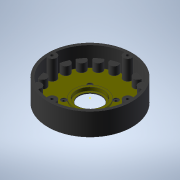
# Autodesk Inventor part: Część8
Saved by Autodesk Inventor 2021 (Build 250183000, 183)
## iProperties
Created: 2022-08-30
Part Number: Część8
Material: Ogólny
Document SubType Name: Modeling
Designer: MicnedSQ
Density: 1 g/cm^3
Appearance: Domyślna
Author: MicnedSQ
## iProperties of the stored document _Drukowanie 3D.ipt
Created: 2022-09-01
Part Number: _Drukowanie 3D
Material: Ogólny
Document SubType Name: Modeling
Designer: MicnedSQ
Density: 1 g/cm^3
Appearance: Domyślna
Author: MicnedSQ
Autodesk Inventor part; units mm, degrees
ref_plane "YZ Plane" through (0, 0, 0) normal (1, 0, 0) x (0, 1, 0)
ref_plane "XZ Plane" through (0, 0, 0) normal (0, 1, 0) x (-1, 0, 0)
ref_plane "XY Plane" through (0, 0, 0) normal (0, 0, 1) x (1, 0, 0)
sketch "Szkic1" plane through (0, 0, 0) normal (0, 1, 0) x (-1, 0, 0)
  circle A0 centre (0, 0) radius 50
  dimension "d1" = 100
  constraints: 1 centre point
  measures "d1" diameter of A0
extrude "Wyciągnięcie proste1" add sketch "Szkic1" along normal blind 5
sketch "Szkic2" plane through (0, 5, 0) normal (0, 1, 0) x (1, 0, 0)
  circle A0 centre (0, 0) radius 13.5
  dimension "d4" = 27
  constraints: 1 centre point, 1 coincident
  measures "d4" diameter of A0
extrude "Wyciągnięcie proste2" cut sketch "Szkic2" against normal through all
sketch "Szkic3" plane through (0, 5, 0) normal (0, 1, 0) x (1, 0, 0)
  circle A0 centre (0, 0) radius 16.1
  dimension "d7" = 32.2
  constraints: 1 centre point, 1 coincident
  measures "d7" diameter of A0
extrude "Wyciągnięcie proste3" cut sketch "Szkic3" against normal blind 4
sketch "Szkic4" plane through (0, 5, 0) normal (0, 1, 0) x (1, 0, 0)
  point P0 (0, 0)
sketch "Szkic5" plane through (0, 5, 0) normal (0, 1, 0) x (1, 0, 0)
  circle A0 centre (0, 0) radius 50
  circle A1 centre (0, 0) radius 50 projected
  circle A2 centre (0, 0) radius 43
  dimension "d10" = 86
  dimension "d78" = 100
  constraints: 2 centre point, 2 coincident
  measures "d10" diameter of A2
  measures "d78" diameter of A0
extrude "Wyciągnięcie proste4" add sketch "Szkic5" along normal blind 18.5
sketch "Szkic7" plane through (0, 5, 0) normal (0, 1, 0) x (1, 0, 0)
  circle A0 centre (-15.6, 15.6) radius 3
  point P0 (0, 0)
  dimension "d19" = 15.6
  dimension "d20" = 15.6
  dimension "d21" = 6
  constraints: 1 centre point, 1 coincident
  measures "d19" horizontal distance of point (0, 0) point (-15.6, 15.6)
  measures "d20" horizontal distance of point (0, 0) point (-15.6, 15.6)
  measures "d21" diameter of A0
extrude "Wyciągnięcie proste6" cut sketch "Szkic7" against normal blind 3
sketch "Szkic8" plane through (-15.6, 2, -15.6) normal (0, 1, 0) x (1, 0, 0)
  circle A0 centre (0, 0) radius 3 projected
  circle A1 centre (0, 0) radius 1.6
  point P0 (15.6, -15.6)
  dimension "d24" = 3.2
  constraints: 1 centre point, 1 coincident
  measures "d24" diameter of A1
extrude "Wyciągnięcie proste7" cut sketch "Szkic8" against normal blind 3 contours A1
pattern_circular "Szyk kołowy2" count 4 over 360 about axis through (0, 5, 0) along (0, -1, 0) of "Wyciągnięcie proste6", "Wyciągnięcie proste7"
sketch "Szkic10" plane through (0, 5, 0) normal (0, 1, 0) x (1, 0, 0)
  circle A0 centre (0, 0) radius 19.0617
  circle A1 centre (15.6, 15.6) radius 3 projected
  circle A2 centre (0, 0) radius 43 projected
  circle A3 centre (0, 0) radius 43 projected
  arc A4 (-28.7568, 31.9695) -> (-21.5185, 37.2284) centre (-26.4503, 36.4058) ccw projected
  arc A5 (-28.7568, 31.9695) -> (-21.5185, 37.2284) centre (-26.4503, 36.4058) ccw projected
  circle A6 centre (0, 0) radius 50 projected
  circle A7 centre (0, 0) radius 43 projected
  point P0 (-28.7568, 31.9695)
  point P1 (13.4787, 13.4787)
  point P2 (-21.5185, 37.2284)
  point P3 (-28.7568, 31.9695)
  point P4 (43, 0)
  point P5 (-28.7568, 31.9695)
  constraints: 1 centre point, 1 tangent
extrude "Wyciągnięcie proste9" cut sketch "Szkic10" against normal blind 2 contours A2 A4 | A4 A2
sketch "Szkic22" plane through (0, 23.5, 0) normal (0, 1, 0) x (1, 0, 0)
  circle A0 centre (0, 0) radius 47
  circle A1 centre (0, 0) radius 16.1 projected
  circle A2 centre (0, 0) radius 43
  dimension "d79" = 94
  constraints: 2 centre point, 2 coincident
  measures "d79" diameter of A0
extrude "Wyciągnięcie proste17" cut sketch "Szkic22" against normal up to surface (20.5 mm away) contours A0
sketch "Szkic24" plane through (0, 3, 0) normal (0, 1, 0) x (1, 0, 0)
  circle A0 centre (0, 45) radius 5
  point P0 (0, 0)
  dimension "d85" = 10
  constraints: 1 centre point
  measures "d85" diameter of A0
extrude "Wyciągnięcie proste18" add sketch "Szkic24" along normal blind 10
pattern_circular "Szyk kołowy6" count 20 over 360 about axis through (0, 23.5, 0) along (0, -1, 0) of "Wyciągnięcie proste18"
sketch "Szkic26" plane through (0, 13, 0) normal (0, 1, 0) x (1, 0, 0)
  arc A0 (-4.6775, 46.7667) -> (4.6775, 46.7667) centre (0, 45) ccw projected
  arc A1 (-4.6775, 46.7667) -> (4.6775, 46.7667) centre (0, 45) ccw
  arc A2 (4.6775, 46.7667) -> (-4.6775, 46.7667) centre (0, 0) ccw
  arc A3 (-46.7667, 4.6775) -> (-46.7667, -4.6775) centre (0, 0) ccw
  arc A4 (-46.7667, -4.6775) -> (-46.7667, 4.6775) centre (-45, 0) ccw
  arc A5 (-4.6775, -46.7667) -> (4.6775, -46.7667) centre (0, 0) ccw
  arc A6 (4.6775, -46.7667) -> (-4.6775, -46.7667) centre (0, -45) ccw
  arc A7 (46.7667, -4.6775) -> (46.7667, 4.6775) centre (0, 0) ccw
  arc A8 (46.7667, 4.6775) -> (46.7667, -4.6775) centre (45, 0) ccw
  point P0 (4.6775, 46.7667)
  point P1 (-4.6775, 46.7667)
  dimension "d96" = 360
  constraints: 16 point on circle, 8 centre point, 4 coincident, 23 other
extrude "Wyciągnięcie proste19" add sketch "Szkic26" along normal up to surface (10.5 mm away)
sketch "Szkic27" plane through (0, 23.5, 0) normal (0, 1, 0) x (1, 0, 0)
  arc A0 (-4.6775, 46.7667) -> (4.6775, 46.7667) centre (0, 45) ccw projected
  circle A1 centre (0, 45) radius 1.95
  point P0 (0, 0)
  dimension "d98" = 3.9
  constraints: 1 centre point, 1 coincident
  measures "d98" diameter of A1
extrude "Wyciągnięcie proste20" cut sketch "Szkic27" against normal blind 6
pattern_circular "Szyk kołowy7" count 4 over 360 about axis through (0, 0, 0) along (0, 1, 0) of "Wyciągnięcie proste20"
sketch "Szkic28" plane through (0, 23.5, 0) normal (0, 1, 0) x (1, 0, 0)
  circle A0 centre (0, 0) radius 50
  circle A1 centre (0, 45) radius 1.95 projected
  circle A2 centre (0, 45) radius 1.95
  arc A3 (-4.6775, 46.7667) -> (4.6775, 46.7667) centre (0, 45) ccw
  arc A4 (-46.7667, -4.6775) -> (-46.7667, 4.6775) centre (-45, 0) ccw
  circle A5 centre (-45, 0) radius 1.95
  arc A6 (4.6775, -46.7667) -> (-4.6775, -46.7667) centre (0, -45) ccw
  circle A7 centre (0, -45) radius 1.95
  arc A8 (46.7667, 4.6775) -> (46.7667, -4.6775) centre (45, 0) ccw
  circle A9 centre (45, 0) radius 1.95
  arc A10 (-4.6775, 46.7667) -> (-46.7667, 4.6775) centre (0, 0) ccw
  arc A11 (46.7667, 4.6775) -> (4.6775, 46.7667) centre (0, 0) ccw
  arc A12 (-46.7667, -4.6775) -> (-4.6775, -46.7667) centre (0, 0) ccw
  arc A13 (4.6775, -46.7667) -> (46.7667, -4.6775) centre (0, 0) ccw
  dimension "d106" = 360
  constraints: 16 point on circle, 13 centre point, 7 coincident, 25 other
extrude "Wyciągnięcie proste21" add sketch "Szkic28" along normal blind 3
